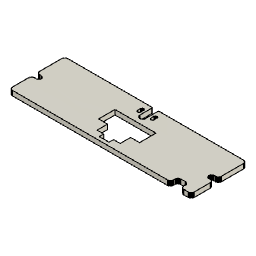
Frame Cover Plate (Autodesk Fusion 360 design; units mm, degrees)
Autodesk Fusion 360 part; units mm, degrees
note: some values were not read from the file. Set by a fixed rule: which sketch regions a step uses.
(part 1 of 3)
sketch "Sketch1" plane through (0, 0, 0) normal (0, 0, 1) x (1, 0, 0) in component "Cover"
  line L0 (69.0119, 5.3264) -> (64.5119, 5.3264)
  line L1 (47.5119, 23.3264) -> (47.5119, 12.3264)
  line L2 (69.0119, 12.3264) -> (69.0119, 5.3264)
  line L3 (75.0119, 12.3264) -> (69.0119, 12.3264)
  line L4 (64.5119, 5.3264) -> (64.5119, 2.3264)
  line L5 (53.5119, 12.3264) -> (53.5119, 5.3264)
  line L6 (64.5119, 2.3264) -> (58.0119, 2.3264)
  line L7 (47.5119, 23.3264) -> (75.0119, 23.3264)
  line L8 (47.5119, 12.3264) -> (53.5119, 12.3264)
  line L9 (58.0119, 2.3264) -> (58.0119, 5.3264)
  line L10 (75.0119, 23.3264) -> (75.0119, 12.3264)
  line L11 (53.5119, 5.3264) -> (58.0119, 5.3264)
  arc A0 (3.7523, 14.957) -> (3.7573, 14.957) centre (3.7548, 14.957) ccw
  arc A1 (3.0339, 14.805) -> (3.0389, 14.805) centre (3.0364, 14.805) ccw
  line L12 (0.8037, 14.387) -> (1.0239, 14.534)
  arc A2 (1.0214, 14.534) -> (1.0264, 14.534) centre (1.0239, 14.534) ccw
  arc A3 (1.0264, 14.534) -> (1.0214, 14.534) centre (1.0239, 14.534) ccw
  line L13 (0.6045, 14.212) -> (0.8037, 14.387)
  arc A4 (1.264, 14.651) -> (1.259, 14.651) centre (1.2615, 14.651) ccw
  arc A5 (0.602, 14.212) -> (0.607, 14.212) centre (0.6045, 14.212) ccw
  line L14 (2.0364, 14.805) -> (3.0364, 14.805)
  arc A6 (1.264, 14.651) -> (1.259, 14.651) centre (1.2615, 14.651) ccw
  arc A7 (0.607, 14.212) -> (0.602, 14.212) centre (0.6045, 14.212) ccw
  arc A8 (2.0339, 14.805) -> (2.0389, 14.805) centre (2.0364, 14.805) ccw
  arc A9 (0.8012, 14.387) -> (0.8062, 14.387) centre (0.8037, 14.387) ccw
  arc A10 (3.043, 14.801) -> (3.048, 14.801) centre (3.0455, 14.801) ccw
  arc A11 (1.5098, 14.736) -> (1.5148, 14.736) centre (1.5123, 14.736) ccw
  line L15 (0.4299, 14.013) -> (0.6045, 14.212)
  arc A12 (0.8012, 14.387) -> (0.8062, 14.387) centre (0.8037, 14.387) ccw
  arc A13 (3.285, 14.818) -> (3.28, 14.818) centre (3.2825, 14.818) ccw
  arc A14 (0.4324, 14.013) -> (0.4274, 14.013) centre (0.4299, 14.013) ccw
  arc A15 (0.8062, 14.387) -> (0.8012, 14.387) centre (0.8037, 14.387) ccw
  arc A16 (0.4274, 14.013) -> (0.4324, 14.013) centre (0.4299, 14.013) ccw
  line L16 (3.5236, 14.871) -> (3.7548, 14.957)
  arc A17 (3.048, 14.801) -> (3.043, 14.801) centre (3.0455, 14.801) ccw
  arc A18 (3.043, 14.801) -> (3.048, 14.801) centre (3.0455, 14.801) ccw
  arc A19 (0.168, 13.555) -> (0.163, 13.555) centre (0.1655, 13.555) ccw
  arc A20 (0.607, 0.598) -> (0.602, 0.598) centre (0.6045, 0.598) ccw
  arc A21 (0.2852, 1.018) -> (0.2802, 1.018) centre (0.2827, 1.018) ccw
  arc A22 (1.7696, 14.788) -> (1.7746, 14.788) centre (1.7721, 14.788) ccw
  arc A23 (3.048, 14.801) -> (3.043, 14.801) centre (3.0455, 14.801) ccw
  arc A24 (0.0089, 12.78) -> (0.0139, 12.78) centre (0.0114, 12.78) ccw
  line L17 (3.7548, 14.957) -> (3.9714, 15.075)
  line L18 (3.2825, 14.818) -> (3.5236, 14.871)
  line L19 (1.0239, 14.534) -> (1.2615, 14.651)
  arc A25 (1.0264, 14.534) -> (1.0214, 14.534) centre (1.0239, 14.534) ccw
  line L20 (3.0455, 14.801) -> (3.2825, 14.818)
  arc A26 (3.0389, 14.805) -> (3.0339, 14.805) centre (3.0364, 14.805) ccw
  arc A27 (3.7573, 14.957) -> (3.7523, 14.957) centre (3.7548, 14.957) ccw
  arc A28 (3.5261, 14.871) -> (3.5211, 14.871) centre (3.5236, 14.871) ccw
  arc A29 (0.4274, 0.797) -> (0.4324, 0.797) centre (0.4299, 0.797) ccw
  arc A30 (4.1714, 15.223) -> (4.1664, 15.223) centre (4.1689, 15.223) ccw
  arc A31 (3.285, 14.818) -> (3.28, 14.818) centre (3.2825, 14.818) ccw
  arc A32 (1.0214, 14.534) -> (1.0264, 14.534) centre (1.0239, 14.534) ccw
  arc A33 (1.7746, 14.788) -> (1.7696, 14.788) centre (1.7721, 14.788) ccw
  arc A34 (0.602, 14.212) -> (0.607, 14.212) centre (0.6045, 14.212) ccw
  arc A35 (0.0262, 13.044) -> (0.0312, 13.044) centre (0.0287, 13.044) ccw
  line L21 (3.0364, 14.805) -> (3.0455, 14.801)
  arc A36 (0.2852, 13.793) -> (0.2802, 13.793) centre (0.2827, 13.793) ccw
  arc A37 (0.163, 13.555) -> (0.168, 13.555) centre (0.1655, 13.555) ccw
  arc A38 (0.4324, 0.797) -> (0.4274, 0.797) centre (0.4299, 0.797) ccw
  arc A39 (3.0339, 14.805) -> (3.0389, 14.805) centre (3.0364, 14.805) ccw
  arc A40 (0.4324, 0.797) -> (0.4274, 0.797) centre (0.4299, 0.797) ccw
  line L22 (0.0114, 2.03) -> (0.0114, 12.78)
  line L23 (0.6045, 0.598) -> (0.8037, 0.423)
  arc A41 (3.9739, 15.075) -> (3.9689, 15.075) centre (3.9714, 15.075) ccw
  arc A42 (3.0389, 14.805) -> (3.0339, 14.805) centre (3.0364, 14.805) ccw
  arc A43 (3.9689, 15.075) -> (3.9739, 15.075) centre (3.9714, 15.075) ccw
  arc A44 (2.0339, 14.805) -> (2.0389, 14.805) centre (2.0364, 14.805) ccw
  arc A45 (3.28, 14.818) -> (3.285, 14.818) centre (3.2825, 14.818) ccw
  line L24 (1.5123, 14.736) -> (1.7721, 14.788)
  arc A46 (2.0389, 14.805) -> (2.0339, 14.805) centre (2.0364, 14.805) ccw
  arc A47 (3.28, 14.818) -> (3.285, 14.818) centre (3.2825, 14.818) ccw
  line L25 (1.7721, 14.788) -> (2.0364, 14.805)
  arc A48 (0.602, 0.598) -> (0.607, 0.598) centre (0.6045, 0.598) ccw
  arc A49 (0.0312, 13.044) -> (0.0262, 13.044) centre (0.0287, 13.044) ccw
  line L26 (0.4299, 0.797) -> (0.6045, 0.598)
  arc A50 (0.168, 1.255) -> (0.163, 1.255) centre (0.1655, 1.255) ccw
  arc A51 (0.607, 14.212) -> (0.602, 14.212) centre (0.6045, 14.212) ccw
  arc A52 (0.0139, 12.78) -> (0.0089, 12.78) centre (0.0114, 12.78) ccw
  arc A53 (0.0779, 1.506) -> (0.0829, 1.506) centre (0.0804, 1.506) ccw
  arc A54 (0.602, 0.598) -> (0.607, 0.598) centre (0.6045, 0.598) ccw
  line L27 (0.1655, 1.255) -> (0.2827, 1.018)
  arc A55 (1.7696, 14.788) -> (1.7746, 14.788) centre (1.7721, 14.788) ccw
  arc A56 (3.5211, 14.871) -> (3.5261, 14.871) centre (3.5236, 14.871) ccw
  arc A57 (1.5148, 14.736) -> (1.5098, 14.736) centre (1.5123, 14.736) ccw
  arc A58 (0.0089, 12.78) -> (0.0139, 12.78) centre (0.0114, 12.78) ccw
  arc A59 (0.4324, 14.013) -> (0.4274, 14.013) centre (0.4299, 14.013) ccw
  line L28 (0.2827, 13.793) -> (0.4299, 14.013)
  arc A60 (3.7523, 14.957) -> (3.7573, 14.957) centre (3.7548, 14.957) ccw
  arc A61 (0.4274, 0.797) -> (0.4324, 0.797) centre (0.4299, 0.797) ccw
  arc A62 (3.5211, 14.871) -> (3.5261, 14.871) centre (3.5236, 14.871) ccw
  arc A63 (3.5261, 14.871) -> (3.5211, 14.871) centre (3.5236, 14.871) ccw
  arc A64 (0.2802, 1.018) -> (0.2852, 1.018) centre (0.2827, 1.018) ccw
  line L29 (1.0239, 0.276) -> (1.2615, 0.159)
  arc A65 (0.0262, 1.766) -> (0.0312, 1.766) centre (0.0287, 1.766) ccw
  line L30 (0.0804, 1.506) -> (0.1655, 1.255)
  arc A66 (106.8089, 0.159) -> (106.8139, 0.159) centre (106.8114, 0.159) ccw
  line L31 (106.8114, 0.159) -> (107.0484, 0.276)
  line L32 (1.7721, 0.022) -> (2.0364, 0.005)
  arc A67 (107.6459, 0.797) -> (107.6409, 0.797) centre (107.6434, 0.797) ccw
  arc A68 (106.8139, 0.159) -> (106.8089, 0.159) centre (106.8114, 0.159) ccw
  arc A69 (1.0214, 0.276) -> (1.0264, 0.276) centre (1.0239, 0.276) ccw
  arc A70 (0.168, 13.555) -> (0.163, 13.555) centre (0.1655, 13.555) ccw
  line L33 (0.0287, 1.766) -> (0.0804, 1.506)
  arc A71 (0.163, 1.255) -> (0.168, 1.255) centre (0.1655, 1.255) ccw
  arc A72 (0.0139, 2.03) -> (0.0089, 2.03) centre (0.0114, 2.03) ccw
  arc A73 (0.168, 1.255) -> (0.163, 1.255) centre (0.1655, 1.255) ccw
  arc A74 (0.0829, 13.304) -> (0.0779, 13.304) centre (0.0804, 13.304) ccw
  arc A75 (0.2802, 13.793) -> (0.2852, 13.793) centre (0.2827, 13.793) ccw
  arc A76 (0.0779, 1.506) -> (0.0829, 1.506) centre (0.0804, 1.506) ccw
  line L34 (0.0114, 12.78) -> (0.0287, 13.044)
  arc A77 (0.163, 1.255) -> (0.168, 1.255) centre (0.1655, 1.255) ccw
  line L35 (0.0287, 13.044) -> (0.0804, 13.304)
  line L36 (0.1655, 13.555) -> (0.2827, 13.793)
  arc A78 (0.0139, 2.03) -> (0.0089, 2.03) centre (0.0114, 2.03) ccw
  arc A79 (0.0312, 13.044) -> (0.0262, 13.044) centre (0.0287, 13.044) ccw
  arc A80 (0.0779, 13.304) -> (0.0829, 13.304) centre (0.0804, 13.304) ccw
  arc A81 (0.0312, 1.766) -> (0.0262, 1.766) centre (0.0287, 1.766) ccw
  arc A82 (0.0312, 1.766) -> (0.0262, 1.766) centre (0.0287, 1.766) ccw
  line L37 (0.2827, 1.018) -> (0.4299, 0.797)
  arc A83 (0.0089, 2.03) -> (0.0139, 2.03) centre (0.0114, 2.03) ccw
  arc A84 (0.2802, 13.793) -> (0.2852, 13.793) centre (0.2827, 13.793) ccw
  arc A85 (107.4709, 0.598) -> (107.4659, 0.598) centre (107.4684, 0.598) ccw
  arc A86 (1.0264, 0.276) -> (1.0214, 0.276) centre (1.0239, 0.276) ccw
  arc A87 (2.0389, 0.005) -> (2.0339, 0.005) centre (2.0364, 0.005) ccw
  arc A88 (0.2852, 1.018) -> (0.2802, 1.018) centre (0.2827, 1.018) ccw
  arc A89 (0.0829, 1.506) -> (0.0779, 1.506) centre (0.0804, 1.506) ccw
  arc A90 (0.8012, 0.423) -> (0.8062, 0.423) centre (0.8037, 0.423) ccw
  arc A91 (1.7696, 0.022) -> (1.7746, 0.022) centre (1.7721, 0.022) ccw
  arc A92 (0.2852, 13.793) -> (0.2802, 13.793) centre (0.2827, 13.793) ccw
  arc A93 (106.2979, 0.022) -> (106.3029, 0.022) centre (106.3004, 0.022) ccw
  arc A94 (1.264, 0.159) -> (1.259, 0.159) centre (1.2615, 0.159) ccw
  arc A95 (1.5098, 0.074) -> (1.5148, 0.074) centre (1.5123, 0.074) ccw
  line L38 (107.6434, 0.797) -> (107.7904, 1.018)
  arc A96 (1.7746, 0.022) -> (1.7696, 0.022) centre (1.7721, 0.022) ccw
  arc A97 (0.0262, 13.044) -> (0.0312, 13.044) centre (0.0287, 13.044) ccw
  arc A98 (0.0139, 12.78) -> (0.0089, 12.78) centre (0.0114, 12.78) ccw
  line L39 (0.0114, 2.03) -> (0.0287, 1.766)
  arc A99 (0.0829, 13.304) -> (0.0779, 13.304) centre (0.0804, 13.304) ccw
  arc A100 (0.0089, 2.03) -> (0.0139, 2.03) centre (0.0114, 2.03) ccw
  line L40 (1.5123, 0.074) -> (1.7721, 0.022)
  arc A101 (0.163, 13.555) -> (0.168, 13.555) centre (0.1655, 13.555) ccw
  arc A102 (0.4274, 14.013) -> (0.4324, 14.013) centre (0.4299, 14.013) ccw
  arc A103 (106.3029, 0.022) -> (106.2979, 0.022) centre (106.3004, 0.022) ccw
  arc A104 (106.5579, 0.074) -> (106.5629, 0.074) centre (106.5604, 0.074) ccw
  arc A105 (0.0779, 13.304) -> (0.0829, 13.304) centre (0.0804, 13.304) ccw
  arc A106 (1.259, 0.159) -> (1.264, 0.159) centre (1.2615, 0.159) ccw
  arc A107 (1.0264, 0.276) -> (1.0214, 0.276) centre (1.0239, 0.276) ccw
  arc A108 (1.5148, 0.074) -> (1.5098, 0.074) centre (1.5123, 0.074) ccw
  arc A109 (106.8089, 0.159) -> (106.8139, 0.159) centre (106.8114, 0.159) ccw
  arc A110 (0.2802, 1.018) -> (0.2852, 1.018) centre (0.2827, 1.018) ccw
  line L41 (0.0804, 13.304) -> (0.1655, 13.555)
  arc A111 (0.0829, 1.506) -> (0.0779, 1.506) centre (0.0804, 1.506) ccw
  arc A112 (0.0262, 1.766) -> (0.0312, 1.766) centre (0.0287, 1.766) ccw
  arc A113 (106.0389, 0.005) -> (106.0339, 0.005) centre (106.0364, 0.005) ccw
  arc A114 (1.7746, 0.022) -> (1.7696, 0.022) centre (1.7721, 0.022) ccw
  line L42 (2.0364, 0.005) -> (106.0364, 0.005)
  line L43 (108.0444, 1.766) -> (108.0614, 2.03)
  line L44 (108.0574, 3.039) -> (108.0744, 3.288)
  arc A115 (108.2049, 3.787) -> (108.2099, 3.787) centre (108.2074, 3.787) ccw
  arc A116 (0.8012, 0.423) -> (0.8062, 0.423) centre (0.8037, 0.423) ccw
  arc A117 (107.6459, 0.797) -> (107.6409, 0.797) centre (107.6434, 0.797) ccw
  line L45 (106.0364, 0.005) -> (106.3004, 0.022)
  line L46 (107.2694, 0.423) -> (107.4684, 0.598)
  arc A118 (2.0389, 0.005) -> (2.0339, 0.005) centre (2.0364, 0.005) ccw
  arc A119 (106.8139, 0.159) -> (106.8089, 0.159) centre (106.8114, 0.159) ccw
  arc A120 (107.0459, 0.276) -> (107.0509, 0.276) centre (107.0484, 0.276) ccw
  line L47 (106.5604, 0.074) -> (106.8114, 0.159)
  arc A121 (107.4709, 0.598) -> (107.4659, 0.598) centre (107.4684, 0.598) ccw
  arc A122 (107.2719, 0.423) -> (107.2669, 0.423) centre (107.2694, 0.423) ccw
  arc A123 (106.0389, 0.005) -> (106.0339, 0.005) centre (106.0364, 0.005) ccw
  arc A124 (1.5148, 0.074) -> (1.5098, 0.074) centre (1.5123, 0.074) ccw
  line L48 (106.3004, 0.022) -> (106.5604, 0.074)
  arc A125 (107.2669, 0.423) -> (107.2719, 0.423) centre (107.2694, 0.423) ccw
  line L49 (0.8037, 0.423) -> (1.0239, 0.276)
  arc A126 (107.9949, 1.506) -> (107.9899, 1.506) centre (107.9924, 1.506) ccw
  arc A127 (108.1269, 3.542) -> (108.1219, 3.542) centre (108.1244, 3.542) ccw
  arc A128 (1.5098, 0.074) -> (1.5148, 0.074) centre (1.5123, 0.074) ccw
  arc A129 (0.607, 0.598) -> (0.602, 0.598) centre (0.6045, 0.598) ccw
  arc A130 (107.4659, 0.598) -> (107.4709, 0.598) centre (107.4684, 0.598) ccw
  arc A131 (106.2979, 0.022) -> (106.3029, 0.022) centre (106.3004, 0.022) ccw
  arc A132 (106.5629, 0.074) -> (106.5579, 0.074) centre (106.5604, 0.074) ccw
  arc A133 (107.6409, 0.797) -> (107.6459, 0.797) centre (107.6434, 0.797) ccw
  line L50 (1.2615, 0.159) -> (1.5123, 0.074)
  arc A134 (1.259, 0.159) -> (1.264, 0.159) centre (1.2615, 0.159) ccw
  arc A135 (0.8062, 0.423) -> (0.8012, 0.423) centre (0.8037, 0.423) ccw
  arc A136 (0.8062, 0.423) -> (0.8012, 0.423) centre (0.8037, 0.423) ccw
  arc A137 (108.0599, 3.039) -> (108.0549, 3.039) centre (108.0574, 3.039) ccw
  arc A138 (1.7696, 0.022) -> (1.7746, 0.022) centre (1.7721, 0.022) ccw
  arc A139 (2.0339, 0.005) -> (2.0389, 0.005) centre (2.0364, 0.005) ccw
  line L51 (107.4684, 0.598) -> (107.6434, 0.797)
  arc A140 (106.3029, 0.022) -> (106.2979, 0.022) centre (106.3004, 0.022) ccw
  arc A141 (106.5629, 0.074) -> (106.5579, 0.074) centre (106.5604, 0.074) ccw
  arc A142 (107.6409, 0.797) -> (107.6459, 0.797) centre (107.6434, 0.797) ccw
  arc A143 (1.0214, 0.276) -> (1.0264, 0.276) centre (1.0239, 0.276) ccw
  arc A144 (108.0469, 1.766) -> (108.0419, 1.766) centre (108.0444, 1.766) ccw
  line L52 (108.0574, 3.039) -> (108.0614, 3.03)
  arc A145 (106.0339, 0.005) -> (106.0389, 0.005) centre (106.0364, 0.005) ccw
  arc A146 (106.5579, 0.074) -> (106.5629, 0.074) centre (106.5604, 0.074) ccw
  arc A147 (108.0719, 3.288) -> (108.0769, 3.288) centre (108.0744, 3.288) ccw
  arc A148 (108.2099, 3.787) -> (108.2049, 3.787) centre (108.2074, 3.787) ccw
  arc A149 (107.4659, 0.598) -> (107.4709, 0.598) centre (107.4684, 0.598) ccw
  arc A150 (107.7879, 1.018) -> (107.7929, 1.018) centre (107.7904, 1.018) ccw
  arc A151 (108.0469, 1.766) -> (108.0419, 1.766) centre (108.0444, 1.766) ccw
  arc A152 (108.0719, 3.288) -> (108.0769, 3.288) centre (108.0744, 3.288) ccw
  arc A153 (106.0339, 0.005) -> (106.0389, 0.005) centre (106.0364, 0.005) ccw
  arc A154 (107.0509, 0.276) -> (107.0459, 0.276) centre (107.0484, 0.276) ccw
  arc A155 (1.264, 0.159) -> (1.259, 0.159) centre (1.2615, 0.159) ccw
  arc A156 (2.0339, 0.005) -> (2.0389, 0.005) centre (2.0364, 0.005) ccw
  arc A157 (65.9959, 29.6125) -> (65.9909, 29.6125) centre (65.9934, 29.6125) ccw
  arc A158 (64.5779, 30.1597) -> (64.5829, 30.1597) centre (64.5804, 30.1597) ccw
  line L53 (65.6314, 29.5094) -> (65.8174, 29.5441)
  arc A159 (65.9909, 29.6125) -> (65.9959, 29.6125) centre (65.9934, 29.6125) ccw
  arc A160 (64.5829, 30.1597) -> (64.5779, 30.1597) centre (64.5804, 30.1597) ccw
  arc A161 (64.7819, 29.8395) -> (64.7769, 29.8395) centre (64.7794, 29.8395) ccw
  line L54 (64.5114, 32.53) -> (64.5284, 32.7183)
  arc A162 (64.5089, 32.53) -> (64.5139, 32.53) centre (64.5114, 32.53) ccw
  arc A163 (64.5139, 32.53) -> (64.5089, 32.53) centre (64.5114, 32.53) ccw
  arc A164 (64.5259, 32.7183) -> (64.5309, 32.7183) centre (64.5284, 32.7183) ccw
  arc A165 (64.5829, 32.9003) -> (64.5779, 32.9003) centre (64.5804, 32.9003) ccw
  arc A166 (64.5259, 30.3417) -> (64.5309, 30.3417) centre (64.5284, 30.3417) ccw
  line L55 (64.7794, 29.8395) -> (64.9184, 29.712)
  arc A167 (64.5089, 30.53) -> (64.5139, 30.53) centre (64.5114, 30.53) ccw
  line L56 (65.0794, 29.6125) -> (65.2554, 29.5441)
  line L57 (65.8174, 29.5441) -> (65.9934, 29.6125)
  line L58 (64.5114, 30.53) -> (64.5284, 30.3417)
  arc A168 (65.9909, 29.6125) -> (65.9959, 29.6125) centre (65.9934, 29.6125) ccw
  arc A169 (64.5259, 30.3417) -> (64.5309, 30.3417) centre (64.5284, 30.3417) ccw
  arc A170 (66.5419, 32.7183) -> (66.5469, 32.7183) centre (66.5444, 32.7183) ccw
  arc A171 (65.8199, 29.5441) -> (65.8149, 29.5441) centre (65.8174, 29.5441) ccw
  arc A172 (66.1519, 29.712) -> (66.1569, 29.712) centre (66.1544, 29.712) ccw
  arc A173 (65.6339, 29.5094) -> (65.6289, 29.5094) centre (65.6314, 29.5094) ccw
  line L59 (64.9184, 29.712) -> (65.0794, 29.6125)
  arc A174 (65.6339, 29.5094) -> (65.6289, 29.5094) centre (65.6314, 29.5094) ccw
  arc A175 (65.4389, 29.5094) -> (65.4439, 29.5094) centre (65.4414, 29.5094) ccw
  arc A176 (65.0819, 29.6125) -> (65.0769, 29.6125) centre (65.0794, 29.6125) ccw
  arc A177 (64.5089, 32.53) -> (64.5139, 32.53) centre (64.5114, 32.53) ccw
  line L60 (65.9934, 29.6125) -> (66.1544, 29.712)
  arc A178 (65.9959, 29.6125) -> (65.9909, 29.6125) centre (65.9934, 29.6125) ccw
  arc A179 (65.0769, 29.6125) -> (65.0819, 29.6125) centre (65.0794, 29.6125) ccw
  arc A180 (64.9159, 29.712) -> (64.9209, 29.712) centre (64.9184, 29.712) ccw
  arc A181 (64.6679, 29.9904) -> (64.6629, 29.9904) centre (64.6654, 29.9904) ccw
  arc A182 (65.8149, 29.5441) -> (65.8199, 29.5441) centre (65.8174, 29.5441) ccw
  arc A183 (64.5139, 30.53) -> (64.5089, 30.53) centre (64.5114, 30.53) ccw
  arc A184 (64.6629, 29.9904) -> (64.6679, 29.9904) centre (64.6654, 29.9904) ccw
  arc A185 (65.4439, 29.5094) -> (65.4389, 29.5094) centre (65.4414, 29.5094) ccw
  arc A186 (65.8149, 29.5441) -> (65.8199, 29.5441) centre (65.8174, 29.5441) ccw
  arc A187 (64.9209, 29.712) -> (64.9159, 29.712) centre (64.9184, 29.712) ccw
  arc A188 (66.1519, 33.348) -> (66.1569, 33.348) centre (66.1544, 33.348) ccw
  arc A189 (66.5589, 30.53) -> (66.5639, 30.53) centre (66.5614, 30.53) ccw
  arc A190 (66.4949, 32.9003) -> (66.4899, 32.9003) centre (66.4924, 32.9003) ccw
  arc A191 (66.2959, 29.8395) -> (66.2909, 29.8395) centre (66.2934, 29.8395) ccw
  line L61 (66.4924, 30.1597) -> (66.5444, 30.3417)
  line L62 (65.2554, 29.5441) -> (65.4414, 29.5094)
  arc A192 (64.5309, 30.3417) -> (64.5259, 30.3417) centre (64.5284, 30.3417) ccw
  arc A193 (66.1569, 29.712) -> (66.1519, 29.712) centre (66.1544, 29.712) ccw
  arc A194 (65.0819, 29.6125) -> (65.0769, 29.6125) centre (65.0794, 29.6125) ccw
  arc A195 (64.7769, 29.8395) -> (64.7819, 29.8395) centre (64.7794, 29.8395) ccw
  arc A196 (65.4439, 29.5094) -> (65.4389, 29.5094) centre (65.4414, 29.5094) ccw
  arc A197 (65.2579, 29.5441) -> (65.2529, 29.5441) centre (65.2554, 29.5441) ccw
  arc A198 (65.0769, 29.6125) -> (65.0819, 29.6125) centre (65.0794, 29.6125) ccw
  arc A199 (64.6629, 29.9904) -> (64.6679, 29.9904) centre (64.6654, 29.9904) ccw
  arc A200 (65.6289, 29.5094) -> (65.6339, 29.5094) centre (65.6314, 29.5094) ccw
  line L63 (64.5804, 30.1597) -> (64.6654, 29.9904)
  line L64 (66.1544, 29.712) -> (66.2934, 29.8395)
  arc A201 (64.5139, 32.53) -> (64.5089, 32.53) centre (64.5114, 32.53) ccw
  line L65 (65.4414, 29.5094) -> (65.6314, 29.5094)
  arc A202 (65.4389, 29.5094) -> (65.4439, 29.5094) centre (65.4414, 29.5094) ccw
  line L66 (64.6654, 29.9904) -> (64.7794, 29.8395)
  arc A203 (64.7819, 29.8395) -> (64.7769, 29.8395) centre (64.7794, 29.8395) ccw
  arc A204 (66.1519, 29.712) -> (66.1569, 29.712) centre (66.1544, 29.712) ccw
  arc A205 (64.5309, 30.3417) -> (64.5259, 30.3417) centre (64.5284, 30.3417) ccw
  arc A206 (65.6289, 29.5094) -> (65.6339, 29.5094) centre (65.6314, 29.5094) ccw
  arc A207 (64.7769, 29.8395) -> (64.7819, 29.8395) centre (64.7794, 29.8395) ccw
  arc A208 (64.5829, 30.1597) -> (64.5779, 30.1597) centre (64.5804, 30.1597) ccw
  arc A209 (65.2529, 29.5441) -> (65.2579, 29.5441) centre (65.2554, 29.5441) ccw
  arc A210 (64.5779, 30.1597) -> (64.5829, 30.1597) centre (64.5804, 30.1597) ccw
  arc A211 (65.8199, 29.5441) -> (65.8149, 29.5441) centre (65.8174, 29.5441) ccw
  arc A212 (64.6679, 29.9904) -> (64.6629, 29.9904) centre (64.6654, 29.9904) ccw
  arc A213 (65.2529, 29.5441) -> (65.2579, 29.5441) centre (65.2554, 29.5441) ccw
  arc A214 (65.2579, 29.5441) -> (65.2529, 29.5441) centre (65.2554, 29.5441) ccw
  arc A215 (64.9209, 29.712) -> (64.9159, 29.712) centre (64.9184, 29.712) ccw
  line L67 (64.5284, 30.3417) -> (64.5804, 30.1597)
  arc A216 (64.9159, 29.712) -> (64.9209, 29.712) centre (64.9184, 29.712) ccw
  arc A217 (65.9959, 33.4475) -> (65.9909, 33.4475) centre (65.9934, 33.4475) ccw
  arc A218 (66.5639, 30.53) -> (66.5589, 30.53) centre (66.5614, 30.53) ccw
  arc A219 (66.1569, 33.348) -> (66.1519, 33.348) centre (66.1544, 33.348) ccw
  arc A220 (66.2959, 33.2205) -> (66.2909, 33.2205) centre (66.2934, 33.2205) ccw
  arc A221 (65.8199, 33.5159) -> (65.8149, 33.5159) centre (65.8174, 33.5159) ccw
  arc A222 (66.4049, 33.0696) -> (66.4099, 33.0696) centre (66.4074, 33.0696) ccw
  arc A223 (66.2959, 29.8395) -> (66.2909, 29.8395) centre (66.2934, 29.8395) ccw
  arc A224 (66.5589, 30.53) -> (66.5639, 30.53) centre (66.5614, 30.53) ccw
  arc A225 (66.5469, 32.7183) -> (66.5419, 32.7183) centre (66.5444, 32.7183) ccw
  line L68 (65.8174, 33.5159) -> (65.9934, 33.4475)
  arc A226 (66.5589, 32.53) -> (66.5639, 32.53) centre (66.5614, 32.53) ccw
  arc A227 (66.2909, 29.8395) -> (66.2959, 29.8395) centre (66.2934, 29.8395) ccw
  arc A228 (66.4949, 30.1597) -> (66.4899, 30.1597) centre (66.4924, 30.1597) ccw
  arc A229 (66.4949, 30.1597) -> (66.4899, 30.1597) centre (66.4924, 30.1597) ccw
  line L69 (66.5614, 30.53) -> (66.5614, 32.53)
  arc A230 (66.4099, 29.9904) -> (66.4049, 29.9904) centre (66.4074, 29.9904) ccw
  arc A231 (66.2909, 33.2205) -> (66.2959, 33.2205) centre (66.2934, 33.2205) ccw
  line L70 (66.5444, 32.7183) -> (66.5614, 32.53)
  arc A232 (66.5469, 30.3417) -> (66.5419, 30.3417) centre (66.5444, 30.3417) ccw
  arc A233 (66.5419, 30.3417) -> (66.5469, 30.3417) centre (66.5444, 30.3417) ccw
  arc A234 (66.4099, 33.0696) -> (66.4049, 33.0696) centre (66.4074, 33.0696) ccw
  arc A235 (66.5589, 32.53) -> (66.5639, 32.53) centre (66.5614, 32.53) ccw
  arc A236 (66.5469, 32.7183) -> (66.5419, 32.7183) centre (66.5444, 32.7183) ccw
  line L71 (66.1544, 33.348) -> (66.2934, 33.2205)
  arc A237 (120.0389, 37.055) -> (120.0339, 37.055) centre (120.0364, 37.055) ccw
  arc A238 (66.4899, 30.1597) -> (66.4949, 30.1597) centre (66.4924, 30.1597) ccw
  arc A239 (65.8149, 33.5159) -> (65.8199, 33.5159) centre (65.8174, 33.5159) ccw
  arc A240 (66.4049, 29.9904) -> (66.4099, 29.9904) centre (66.4074, 29.9904) ccw
  arc A241 (66.5639, 30.53) -> (66.5589, 30.53) centre (66.5614, 30.53) ccw
  arc A242 (65.9909, 33.4475) -> (65.9959, 33.4475) centre (65.9934, 33.4475) ccw
  line L72 (66.4074, 33.0696) -> (66.4924, 32.9003)
  arc A243 (66.4099, 33.0696) -> (66.4049, 33.0696) centre (66.4074, 33.0696) ccw
  arc A244 (66.5639, 32.53) -> (66.5589, 32.53) centre (66.5614, 32.53) ccw
  arc A245 (66.4899, 32.9003) -> (66.4949, 32.9003) centre (66.4924, 32.9003) ccw
  line L73 (66.5444, 30.3417) -> (66.5614, 30.53)
  arc A246 (66.5419, 32.7183) -> (66.5469, 32.7183) centre (66.5444, 32.7183) ccw
  arc A247 (65.9909, 33.4475) -> (65.9959, 33.4475) centre (65.9934, 33.4475) ccw
  arc A248 (66.5469, 30.3417) -> (66.5419, 30.3417) centre (66.5444, 30.3417) ccw
  arc A249 (66.1519, 33.348) -> (66.1569, 33.348) centre (66.1544, 33.348) ccw
  line L74 (65.9934, 33.4475) -> (66.1544, 33.348)
  arc A250 (66.5639, 32.53) -> (66.5589, 32.53) centre (66.5614, 32.53) ccw
  line L75 (66.4924, 32.9003) -> (66.5444, 32.7183)
  line L76 (66.2934, 33.2205) -> (66.4074, 33.0696)
  arc A251 (66.4949, 32.9003) -> (66.4899, 32.9003) centre (66.4924, 32.9003) ccw
  arc A252 (66.4899, 32.9003) -> (66.4949, 32.9003) centre (66.4924, 32.9003) ccw
  arc A253 (66.4899, 30.1597) -> (66.4949, 30.1597) centre (66.4924, 30.1597) ccw
  arc A254 (66.1569, 29.712) -> (66.1519, 29.712) centre (66.1544, 29.712) ccw
  arc A255 (66.2909, 29.8395) -> (66.2959, 29.8395) centre (66.2934, 29.8395) ccw
  line L77 (66.4074, 29.9904) -> (66.4924, 30.1597)
  arc A256 (66.4099, 29.9904) -> (66.4049, 29.9904) centre (66.4074, 29.9904) ccw
  arc A257 (66.4049, 29.9904) -> (66.4099, 29.9904) centre (66.4074, 29.9904) ccw
  arc A258 (66.1569, 33.348) -> (66.1519, 33.348) centre (66.1544, 33.348) ccw
  arc A259 (66.2959, 33.2205) -> (66.2909, 33.2205) centre (66.2934, 33.2205) ccw
  arc A260 (66.5419, 30.3417) -> (66.5469, 30.3417) centre (66.5444, 30.3417) ccw
  line L78 (66.2934, 29.8395) -> (66.4074, 29.9904)
  arc A261 (65.9959, 33.4475) -> (65.9909, 33.4475) centre (65.9934, 33.4475) ccw
  arc A262 (66.4049, 33.0696) -> (66.4099, 33.0696) centre (66.4074, 33.0696) ccw
  arc A263 (66.2909, 33.2205) -> (66.2959, 33.2205) centre (66.2934, 33.2205) ccw
  line L79 (120.3004, 37.0377) -> (120.5604, 36.986)
  arc A264 (120.2979, 37.0377) -> (120.3029, 37.0377) centre (120.3004, 37.0377) ccw
  arc A265 (63.2069, 36.9405) -> (63.2119, 36.9405) centre (63.2094, 36.9405) ccw
  arc A266 (120.5629, 36.986) -> (120.5579, 36.986) centre (120.5604, 36.986) ccw
  line L80 (120.0364, 37.055) -> (120.3004, 37.0377)
  line L81 (63.3084, 37.003) -> (63.4194, 37.0418)
  arc A267 (62.9999, 28.2604) -> (62.9949, 28.2604) centre (62.9974, 28.2604) ccw
  arc A268 (63.0089, 36.53) -> (63.0139, 36.53) centre (63.0114, 36.53) ccw
  arc A269 (62.9949, 28.2604) -> (62.9999, 28.2604) centre (62.9974, 28.2604) ccw
  line L82 (62.9974, 28.2604) -> (63.0154, 28.5204)
  arc A270 (120.0339, 37.055) -> (120.0389, 37.055) centre (120.0364, 37.055) ccw
  arc A271 (63.1239, 36.8573) -> (63.1289, 36.8573) centre (63.1264, 36.8573) ccw
  arc A272 (63.0129, 28.5204) -> (63.0179, 28.5204) centre (63.0154, 28.5204) ccw
  arc A273 (63.0269, 36.6468) -> (63.0219, 36.6468) centre (63.0244, 36.6468) ccw
  arc A274 (63.0129, 28.5204) -> (63.0179, 28.5204) centre (63.0154, 28.5204) ccw
  arc A275 (63.3059, 37.003) -> (63.3109, 37.003) centre (63.3084, 37.003) ccw
  arc A276 (63.0179, 28.5204) -> (63.0129, 28.5204) centre (63.0154, 28.5204) ccw
  arc A277 (63.4169, 37.0418) -> (63.4219, 37.0418) centre (63.4194, 37.0418) ccw
  arc A278 (63.0089, 36.53) -> (63.0139, 36.53) centre (63.0114, 36.53) ccw
  arc A279 (63.2119, 36.9405) -> (63.2069, 36.9405) centre (63.2094, 36.9405) ccw
  arc A280 (120.3029, 37.0377) -> (120.2979, 37.0377) centre (120.3004, 37.0377) ccw
  line L83 (63.0114, 28.53) -> (63.0114, 36.53)
  arc A281 (63.2119, 36.9405) -> (63.2069, 36.9405) centre (63.2094, 36.9405) ccw
  arc A282 (120.3029, 37.0377) -> (120.2979, 37.0377) centre (120.3004, 37.0377) ccw
  arc A283 (63.1289, 36.8573) -> (63.1239, 36.8573) centre (63.1264, 36.8573) ccw
  arc A284 (63.0659, 36.7578) -> (63.0609, 36.7578) centre (63.0634, 36.7578) ccw
  arc A285 (63.0269, 36.6468) -> (63.0219, 36.6468) centre (63.0244, 36.6468) ccw
  arc A286 (63.0089, 28.53) -> (63.0139, 28.53) centre (63.0114, 28.53) ccw
  arc A287 (120.0389, 37.055) -> (120.0339, 37.055) centre (120.0364, 37.055) ccw
  line L84 (63.0114, 28.53) -> (63.0154, 28.5204)
  arc A288 (63.4219, 37.0418) -> (63.4169, 37.0418) centre (63.4194, 37.0418) ccw
  arc A289 (63.5389, 37.055) -> (63.5339, 37.055) centre (63.5364, 37.055) ccw
  arc A290 (63.2069, 36.9405) -> (63.2119, 36.9405) centre (63.2094, 36.9405) ccw
  arc A291 (63.0609, 36.7578) -> (63.0659, 36.7578) centre (63.0634, 36.7578) ccw
  arc A292 (63.4219, 37.0418) -> (63.4169, 37.0418) centre (63.4194, 37.0418) ccw
  arc A293 (63.0089, 28.53) -> (63.0139, 28.53) centre (63.0114, 28.53) ccw
  line L85 (63.2094, 36.9405) -> (63.3084, 37.003)
  arc A294 (63.5339, 37.055) -> (63.5389, 37.055) centre (63.5364, 37.055) ccw
  arc A295 (63.0219, 36.6468) -> (63.0269, 36.6468) centre (63.0244, 36.6468) ccw
  arc A296 (63.1239, 36.8573) -> (63.1289, 36.8573) centre (63.1264, 36.8573) ccw
  line L86 (63.5364, 37.055) -> (120.0364, 37.055)
  arc A297 (63.4169, 37.0418) -> (63.4219, 37.0418) centre (63.4194, 37.0418) ccw
  arc A298 (63.0179, 28.5204) -> (63.0129, 28.5204) centre (63.0154, 28.5204) ccw
  arc A299 (63.5389, 37.055) -> (63.5339, 37.055) centre (63.5364, 37.055) ccw
  arc A300 (63.3109, 37.003) -> (63.3059, 37.003) centre (63.3084, 37.003) ccw
  arc A301 (63.0609, 36.7578) -> (63.0659, 36.7578) centre (63.0634, 36.7578) ccw
  line L87 (63.4194, 37.0418) -> (63.5364, 37.055)
  arc A302 (63.0139, 36.53) -> (63.0089, 36.53) centre (63.0114, 36.53) ccw
  arc A303 (63.1289, 36.8573) -> (63.1239, 36.8573) centre (63.1264, 36.8573) ccw
  line L88 (63.0634, 36.7578) -> (63.1264, 36.8573)
  arc A304 (63.0219, 36.6468) -> (63.0269, 36.6468) centre (63.0244, 36.6468) ccw
  line L89 (63.0114, 36.53) -> (63.0244, 36.6468)
  line L90 (63.1264, 36.8573) -> (63.2094, 36.9405)
  arc A305 (63.3109, 37.003) -> (63.3059, 37.003) centre (63.3084, 37.003) ccw
  line L91 (63.0244, 36.6468) -> (63.0634, 36.7578)
  arc A306 (63.0139, 28.53) -> (63.0089, 28.53) centre (63.0114, 28.53) ccw
  arc A307 (63.0659, 36.7578) -> (63.0609, 36.7578) centre (63.0634, 36.7578) ccw
  arc A308 (63.0139, 36.53) -> (63.0089, 36.53) centre (63.0114, 36.53) ccw
  arc A309 (63.0139, 28.53) -> (63.0089, 28.53) centre (63.0114, 28.53) ccw
  arc A310 (120.5579, 36.986) -> (120.5629, 36.986) centre (120.5604, 36.986) ccw
  arc A311 (120.2979, 37.0377) -> (120.3029, 37.0377) centre (120.3004, 37.0377) ccw
  arc A312 (63.5339, 37.055) -> (63.5389, 37.055) centre (63.5364, 37.055) ccw
  arc A313 (63.3059, 37.003) -> (63.3109, 37.003) centre (63.3084, 37.003) ccw
  arc A314 (61.9449, 26.7723) -> (61.9499, 26.7723) centre (61.9474, 26.7723) ccw
  line L92 (62.7274, 27.5014) -> (62.8524, 27.7413)
  line L93 (61.4394, 26.5918) -> (61.6994, 26.6647)
  arc A315 (61.4419, 26.5918) -> (61.4369, 26.5918) centre (61.4394, 26.5918) ccw
  line L94 (62.5724, 27.2807) -> (62.7274, 27.5014)
  arc A316 (60.9038, 26.555) -> (60.8988, 26.555) centre (60.9013, 26.555) ccw
  arc A317 (60.376, 26.6647) -> (60.371, 26.6647) centre (60.3735, 26.6647) ccw
  arc A318 (62.1759, 26.9127) -> (62.1809, 26.9127) centre (62.1784, 26.9127) ccw
  arc A319 (61.1689, 26.555) -> (61.1739, 26.555) centre (61.1714, 26.555) ccw
  arc A320 (61.7019, 26.6647) -> (61.6969, 26.6647) centre (61.6994, 26.6647) ccw
  arc A321 (120.0339, 37.055) -> (120.0389, 37.055) centre (120.0364, 37.055) ccw
  arc A322 (62.8499, 27.7413) -> (62.8549, 27.7413) centre (62.8524, 27.7413) ccw
  arc A323 (61.4369, 26.5918) -> (61.4419, 26.5918) centre (61.4394, 26.5918) ccw
  arc A324 (61.1739, 26.555) -> (61.1689, 26.555) centre (61.1714, 26.555) ccw
  arc A325 (61.4419, 26.5918) -> (61.4369, 26.5918) centre (61.4394, 26.5918) ccw
  arc A326 (62.3899, 27.0832) -> (62.3849, 27.0832) centre (62.3874, 27.0832) ccw
  arc A327 (62.9999, 28.2604) -> (62.9949, 28.2604) centre (62.9974, 28.2604) ccw
  arc A328 (62.7299, 27.5014) -> (62.7249, 27.5014) centre (62.7274, 27.5014) ccw
  arc A329 (61.9499, 26.7723) -> (61.9449, 26.7723) centre (61.9474, 26.7723) ccw
  arc A330 (61.1689, 26.555) -> (61.1739, 26.555) centre (61.1714, 26.555) ccw
  arc A331 (62.1809, 26.9127) -> (62.1759, 26.9127) centre (62.1784, 26.9127) ccw
  arc A332 (60.371, 26.6647) -> (60.376, 26.6647) centre (60.3735, 26.6647) ccw
  arc A333 (62.5699, 27.2807) -> (62.5749, 27.2807) centre (62.5724, 27.2807) ccw
  arc A334 (60.8988, 26.555) -> (60.9038, 26.555) centre (60.9013, 26.555) ccw
  arc A335 (60.6311, 26.5918) -> (60.6361, 26.5918) centre (60.6336, 26.5918) ccw
  arc A336 (62.9949, 28.2604) -> (62.9999, 28.2604) centre (62.9974, 28.2604) ccw
  arc A337 (61.1739, 26.555) -> (61.1689, 26.555) centre (61.1714, 26.555) ccw
  line L95 (60.9013, 26.555) -> (61.1714, 26.555)
  arc A338 (62.8499, 27.7413) -> (62.8549, 27.7413) centre (62.8524, 27.7413) ccw
  arc A339 (60.8988, 26.555) -> (60.9038, 26.555) centre (60.9013, 26.555) ccw
  arc A340 (62.1809, 26.9127) -> (62.1759, 26.9127) centre (62.1784, 26.9127) ccw
  arc A341 (62.3849, 27.0832) -> (62.3899, 27.0832) centre (62.3874, 27.0832) ccw
  arc A342 (62.7249, 27.5014) -> (62.7299, 27.5014) centre (62.7274, 27.5014) ccw
  arc A343 (62.3899, 27.0832) -> (62.3849, 27.0832) centre (62.3874, 27.0832) ccw
  arc A344 (62.9399, 27.9959) -> (62.9449, 27.9959) centre (62.9424, 27.9959) ccw
  line L96 (60.3735, 26.6647) -> (60.6336, 26.5918)
  arc A345 (60.6311, 26.5918) -> (60.6361, 26.5918) centre (60.6336, 26.5918) ccw
  line L97 (62.3874, 27.0832) -> (62.5724, 27.2807)
  arc A346 (61.4369, 26.5918) -> (61.4419, 26.5918) centre (61.4394, 26.5918) ccw
  line L98 (62.9424, 27.9959) -> (62.9974, 28.2604)
  line L99 (62.1784, 26.9127) -> (62.3874, 27.0832)
  arc A347 (62.5749, 27.2807) -> (62.5699, 27.2807) centre (62.5724, 27.2807) ccw
  line L100 (61.9474, 26.7723) -> (62.1784, 26.9127)
  arc A348 (62.5699, 27.2807) -> (62.5749, 27.2807) centre (62.5724, 27.2807) ccw
  arc A349 (61.6969, 26.6647) -> (61.7019, 26.6647) centre (61.6994, 26.6647) ccw
  arc A350 (61.7019, 26.6647) -> (61.6969, 26.6647) centre (61.6994, 26.6647) ccw
  line L101 (62.8524, 27.7413) -> (62.9424, 27.9959)
  arc A351 (62.3849, 27.0832) -> (62.3899, 27.0832) centre (62.3874, 27.0832) ccw
  arc A352 (60.6361, 26.5918) -> (60.6311, 26.5918) centre (60.6336, 26.5918) ccw
  arc A353 (61.6969, 26.6647) -> (61.7019, 26.6647) centre (61.6994, 26.6647) ccw
  arc A354 (61.9449, 26.7723) -> (61.9499, 26.7723) centre (61.9474, 26.7723) ccw
  arc A355 (62.5749, 27.2807) -> (62.5699, 27.2807) centre (62.5724, 27.2807) ccw
  arc A356 (62.7299, 27.5014) -> (62.7249, 27.5014) centre (62.7274, 27.5014) ccw
  arc A357 (62.8549, 27.7413) -> (62.8499, 27.7413) centre (62.8524, 27.7413) ccw
  line L102 (60.6336, 26.5918) -> (60.9013, 26.555)
  arc A358 (62.9449, 27.9959) -> (62.9399, 27.9959) centre (62.9424, 27.9959) ccw
  arc A359 (62.7249, 27.5014) -> (62.7299, 27.5014) centre (62.7274, 27.5014) ccw
  arc A360 (61.9499, 26.7723) -> (61.9449, 26.7723) centre (61.9474, 26.7723) ccw
  arc A361 (62.9449, 27.9959) -> (62.9399, 27.9959) centre (62.9424, 27.9959) ccw
  line L103 (61.6994, 26.6647) -> (61.9474, 26.7723)
  arc A362 (60.9038, 26.555) -> (60.8988, 26.555) centre (60.9013, 26.555) ccw
  line L104 (61.1714, 26.555) -> (61.4394, 26.5918)
  arc A363 (62.1759, 26.9127) -> (62.1809, 26.9127) centre (62.1784, 26.9127) ccw
  line L105 (59.1302, 27.9959) -> (59.2207, 27.7413)
  arc A364 (59.0069, 36.7578) -> (59.0119, 36.7578) centre (59.0094, 36.7578) ccw
  arc A365 (59.1327, 27.9959) -> (59.1277, 27.9959) centre (59.1302, 27.9959) ccw
  arc A366 (59.2232, 27.7413) -> (59.2182, 27.7413) centre (59.2207, 27.7413) ccw
  line L106 (59.0482, 36.6468) -> (59.0614, 36.53)
  arc A367 (59.0507, 36.6468) -> (59.0457, 36.6468) centre (59.0482, 36.6468) ccw
  arc A368 (59.0639, 36.53) -> (59.0589, 36.53) centre (59.0614, 36.53) ccw
  arc A369 (59.2232, 27.7413) -> (59.2182, 27.7413) centre (59.2207, 27.7413) ccw
  arc A370 (59.0549, 28.5204) -> (59.0599, 28.5204) centre (59.0574, 28.5204) ccw
  line L107 (59.345, 27.5014) -> (59.5008, 27.2807)
  line L108 (59.0752, 28.2604) -> (59.1302, 27.9959)
  arc A371 (60.6361, 26.5918) -> (60.6311, 26.5918) centre (60.6336, 26.5918) ccw
  arc A372 (59.0599, 28.5204) -> (59.0549, 28.5204) centre (59.0574, 28.5204) ccw
  arc A373 (59.1327, 27.9959) -> (59.1277, 27.9959) centre (59.1302, 27.9959) ccw
  arc A374 (60.1231, 26.7723) -> (60.1281, 26.7723) centre (60.1256, 26.7723) ccw
  line L109 (60.1256, 26.7723) -> (60.3735, 26.6647)
  arc A375 (62.8549, 27.7413) -> (62.8499, 27.7413) centre (62.8524, 27.7413) ccw
  line L110 (59.6852, 27.0832) -> (59.8948, 26.9127)
  arc A376 (62.9399, 27.9959) -> (62.9449, 27.9959) centre (62.9424, 27.9959) ccw
  arc A377 (59.8923, 26.9127) -> (59.8973, 26.9127) centre (59.8948, 26.9127) ccw
  arc A378 (59.0549, 28.5204) -> (59.0599, 28.5204) centre (59.0574, 28.5204) ccw
  arc A379 (60.376, 26.6647) -> (60.371, 26.6647) centre (60.3735, 26.6647) ccw
  arc A380 (60.1281, 26.7723) -> (60.1231, 26.7723) centre (60.1256, 26.7723) ccw
  arc A381 (59.8973, 26.9127) -> (59.8923, 26.9127) centre (59.8948, 26.9127) ccw
  arc A382 (59.1277, 27.9959) -> (59.1327, 27.9959) centre (59.1302, 27.9959) ccw
  line L111 (59.0574, 28.5204) -> (59.0752, 28.2604)
  arc A383 (59.2182, 27.7413) -> (59.2232, 27.7413) centre (59.2207, 27.7413) ccw
  arc A384 (59.8923, 26.9127) -> (59.8973, 26.9127) centre (59.8948, 26.9127) ccw
  arc A385 (59.0589, 28.53) -> (59.0639, 28.53) centre (59.0614, 28.53) ccw
  arc A386 (59.0639, 28.53) -> (59.0589, 28.53) centre (59.0614, 28.53) ccw
  arc A387 (59.1277, 27.9959) -> (59.1327, 27.9959) centre (59.1302, 27.9959) ccw
  arc A388 (59.0589, 36.53) -> (59.0639, 36.53) centre (59.0614, 36.53) ccw
  line L112 (59.2207, 27.7413) -> (59.345, 27.5014)
  arc A389 (59.3475, 27.5014) -> (59.3425, 27.5014) centre (59.345, 27.5014) ccw
  line L113 (59.0094, 36.7578) -> (59.0482, 36.6468)
  arc A390 (59.0589, 28.53) -> (59.0639, 28.53) centre (59.0614, 28.53) ccw
  arc A391 (59.4983, 27.2807) -> (59.5033, 27.2807) centre (59.5008, 27.2807) ccw
  arc A392 (59.4983, 27.2807) -> (59.5033, 27.2807) centre (59.5008, 27.2807) ccw
  arc A393 (59.6827, 27.0832) -> (59.6877, 27.0832) centre (59.6852, 27.0832) ccw
  arc A394 (59.5033, 27.2807) -> (59.4983, 27.2807) centre (59.5008, 27.2807) ccw
  arc A395 (59.0639, 28.53) -> (59.0589, 28.53) centre (59.0614, 28.53) ccw
  line L114 (59.8948, 26.9127) -> (60.1256, 26.7723)
  arc A396 (59.0457, 36.6468) -> (59.0507, 36.6468) centre (59.0482, 36.6468) ccw
  arc A397 (59.0639, 36.53) -> (59.0589, 36.53) centre (59.0614, 36.53) ccw
  line L115 (59.0574, 28.5204) -> (59.0614, 28.53)
  arc A398 (59.0589, 36.53) -> (59.0639, 36.53) centre (59.0614, 36.53) ccw
  arc A399 (59.6877, 27.0832) -> (59.6827, 27.0832) centre (59.6852, 27.0832) ccw
  arc A400 (59.6827, 27.0832) -> (59.6877, 27.0832) centre (59.6852, 27.0832) ccw
  arc A401 (59.0777, 28.2604) -> (59.0727, 28.2604) centre (59.0752, 28.2604) ccw
  arc A402 (59.0599, 28.5204) -> (59.0549, 28.5204) centre (59.0574, 28.5204) ccw
  arc A403 (59.8973, 26.9127) -> (59.8923, 26.9127) centre (59.8948, 26.9127) ccw
  arc A404 (59.3425, 27.5014) -> (59.3475, 27.5014) centre (59.345, 27.5014) ccw
  arc A405 (60.1281, 26.7723) -> (60.1231, 26.7723) centre (60.1256, 26.7723) ccw
  arc A406 (59.5033, 27.2807) -> (59.4983, 27.2807) centre (59.5008, 27.2807) ccw
  line L116 (59.0614, 28.53) -> (59.0614, 36.53)
  arc A407 (59.0119, 36.7578) -> (59.0069, 36.7578) centre (59.0094, 36.7578) ccw
  arc A408 (59.3425, 27.5014) -> (59.3475, 27.5014) centre (59.345, 27.5014) ccw
  arc A409 (59.2182, 27.7413) -> (59.2232, 27.7413) centre (59.2207, 27.7413) ccw
  arc A410 (59.3475, 27.5014) -> (59.3425, 27.5014) centre (59.345, 27.5014) ccw
  line L117 (58.5364, 37.055) -> (58.6532, 37.0418)
  arc A411 (1.5098, 36.986) -> (1.5148, 36.986) centre (1.5123, 36.986) ccw
  arc A412 (58.6507, 37.0418) -> (58.6557, 37.0418) centre (58.6532, 37.0418) ccw
  arc A413 (59.0727, 28.2604) -> (59.0777, 28.2604) centre (59.0752, 28.2604) ccw
  arc A414 (0.4274, 36.2627) -> (0.4324, 36.2627) centre (0.4299, 36.2627) ccw
  line L118 (1.5123, 36.986) -> (1.7721, 37.0377)
  arc A415 (59.0507, 36.6468) -> (59.0457, 36.6468) centre (59.0482, 36.6468) ccw
  arc A416 (2.0339, 37.055) -> (2.0389, 37.055) centre (2.0364, 37.055) ccw
  arc A417 (58.9444, 36.8573) -> (58.9494, 36.8573) centre (58.9469, 36.8573) ccw
  arc A418 (0.8062, 36.6365) -> (0.8012, 36.6365) centre (0.8037, 36.6365) ccw
  arc A419 (58.8612, 36.9405) -> (58.8662, 36.9405) centre (58.8637, 36.9405) ccw
  arc A420 (58.6557, 37.0418) -> (58.6507, 37.0418) centre (58.6532, 37.0418) ccw
  arc A421 (1.0264, 36.7837) -> (1.0214, 36.7837) centre (1.0239, 36.7837) ccw
  arc A422 (58.7617, 37.003) -> (58.7667, 37.003) centre (58.7642, 37.003) ccw
  arc A423 (2.0339, 37.055) -> (2.0389, 37.055) centre (2.0364, 37.055) ccw
  line L119 (0.8037, 36.6365) -> (1.0239, 36.7837)
  arc A424 (1.0214, 36.7837) -> (1.0264, 36.7837) centre (1.0239, 36.7837) ccw
  line L120 (1.7721, 37.0377) -> (2.0364, 37.055)
  arc A425 (59.6877, 27.0832) -> (59.6827, 27.0832) centre (59.6852, 27.0832) ccw
  arc A426 (58.9494, 36.8573) -> (58.9444, 36.8573) centre (58.9469, 36.8573) ccw
  line L121 (58.9469, 36.8573) -> (59.0094, 36.7578)
  arc A427 (1.5098, 36.986) -> (1.5148, 36.986) centre (1.5123, 36.986) ccw
  arc A428 (59.0457, 36.6468) -> (59.0507, 36.6468) centre (59.0482, 36.6468) ccw
  line L122 (2.0364, 37.055) -> (58.5364, 37.055)
  arc A429 (58.9444, 36.8573) -> (58.9494, 36.8573) centre (58.9469, 36.8573) ccw
  line L123 (0.6045, 36.4619) -> (0.8037, 36.6365)
  arc A430 (1.7746, 37.0377) -> (1.7696, 37.0377) centre (1.7721, 37.0377) ccw
  line L124 (1.0239, 36.7837) -> (1.2615, 36.9009)
  arc A431 (58.5389, 37.055) -> (58.5339, 37.055) centre (58.5364, 37.055) ccw
  arc A432 (59.0119, 36.7578) -> (59.0069, 36.7578) centre (59.0094, 36.7578) ccw
  arc A433 (2.0389, 37.055) -> (2.0339, 37.055) centre (2.0364, 37.055) ccw
  arc A434 (59.0727, 28.2604) -> (59.0777, 28.2604) centre (59.0752, 28.2604) ccw
  arc A435 (58.5339, 37.055) -> (58.5389, 37.055) centre (58.5364, 37.055) ccw
  line L125 (0.4299, 36.2627) -> (0.6045, 36.4619)
  line L126 (58.6532, 37.0418) -> (58.7642, 37.003)
  arc A436 (60.1231, 26.7723) -> (60.1281, 26.7723) centre (60.1256, 26.7723) ccw
  arc A437 (59.0777, 28.2604) -> (59.0727, 28.2604) centre (59.0752, 28.2604) ccw
  arc A438 (58.6557, 37.0418) -> (58.6507, 37.0418) centre (58.6532, 37.0418) ccw
  arc A439 (59.0069, 36.7578) -> (59.0119, 36.7578) centre (59.0094, 36.7578) ccw
  arc A440 (60.371, 26.6647) -> (60.376, 26.6647) centre (60.3735, 26.6647) ccw
  arc A441 (0.602, 36.4619) -> (0.607, 36.4619) centre (0.6045, 36.4619) ccw
  arc A442 (58.6507, 37.0418) -> (58.6557, 37.0418) centre (58.6532, 37.0418) ccw
  arc A443 (0.8012, 36.6365) -> (0.8062, 36.6365) centre (0.8037, 36.6365) ccw
  arc A444 (58.9494, 36.8573) -> (58.9444, 36.8573) centre (58.9469, 36.8573) ccw
  arc A445 (1.0214, 36.7837) -> (1.0264, 36.7837) centre (1.0239, 36.7837) ccw
  arc A446 (58.7617, 37.003) -> (58.7667, 37.003) centre (58.7642, 37.003) ccw
  arc A447 (2.0389, 37.055) -> (2.0339, 37.055) centre (2.0364, 37.055) ccw
  line L127 (58.8637, 36.9405) -> (58.9469, 36.8573)
  arc A448 (58.8662, 36.9405) -> (58.8612, 36.9405) centre (58.8637, 36.9405) ccw
  arc A449 (1.5148, 36.986) -> (1.5098, 36.986) centre (1.5123, 36.986) ccw
  line L128 (1.2615, 36.9009) -> (1.5123, 36.986)
  arc A450 (1.259, 36.9009) -> (1.264, 36.9009) centre (1.2615, 36.9009) ccw
  arc A451 (0.8062, 36.6365) -> (0.8012, 36.6365) centre (0.8037, 36.6365) ccw
  line L129 (59.5008, 27.2807) -> (59.6852, 27.0832)
  arc A452 (0.8012, 36.6365) -> (0.8062, 36.6365) centre (0.8037, 36.6365) ccw
  arc A453 (58.5339, 37.055) -> (58.5389, 37.055) centre (58.5364, 37.055) ccw
  arc A454 (1.7746, 37.0377) -> (1.7696, 37.0377) centre (1.7721, 37.0377) ccw
  line L130 (58.7642, 37.003) -> (58.8637, 36.9405)
  arc A455 (58.7667, 37.003) -> (58.7617, 37.003) centre (58.7642, 37.003) ccw
  arc A456 (1.264, 36.9009) -> (1.259, 36.9009) centre (1.2615, 36.9009) ccw
  arc A457 (58.8612, 36.9405) -> (58.8662, 36.9405) centre (58.8637, 36.9405) ccw
  arc A458 (0.607, 36.4619) -> (0.602, 36.4619) centre (0.6045, 36.4619) ccw
  arc A459 (1.7696, 37.0377) -> (1.7746, 37.0377) centre (1.7721, 37.0377) ccw
  arc A460 (1.5148, 36.986) -> (1.5098, 36.986) centre (1.5123, 36.986) ccw
  line L131 (0.2827, 19.2675) -> (0.4299, 19.0473)
  line L132 (0.2827, 36.0425) -> (0.4299, 36.2627)
  arc A461 (0.607, 18.8481) -> (0.602, 18.8481) centre (0.6045, 18.8481) ccw
  arc A462 (1.0264, 36.7837) -> (1.0214, 36.7837) centre (1.0239, 36.7837) ccw
  arc A463 (0.168, 19.5051) -> (0.163, 19.5051) centre (0.1655, 19.5051) ccw
  arc A464 (0.0262, 35.2943) -> (0.0312, 35.2943) centre (0.0287, 35.2943) ccw
  arc A465 (0.0829, 19.7559) -> (0.0779, 19.7559) centre (0.0804, 19.7559) ccw
  arc A466 (0.0312, 35.2943) -> (0.0262, 35.2943) centre (0.0287, 35.2943) ccw
  line L133 (0.0804, 35.5541) -> (0.1655, 35.8049)
  arc A467 (0.168, 35.8049) -> (0.163, 35.8049) centre (0.1655, 35.8049) ccw
  line L134 (0.1655, 19.5051) -> (0.2827, 19.2675)
  line L135 (0.0287, 20.0157) -> (0.0804, 19.7559)
  line L136 (0.0804, 19.7559) -> (0.1655, 19.5051)
  arc A468 (0.2802, 19.2675) -> (0.2852, 19.2675) centre (0.2827, 19.2675) ccw
  arc A469 (0.0262, 20.0157) -> (0.0312, 20.0157) centre (0.0287, 20.0157) ccw
  arc A470 (0.4274, 19.0473) -> (0.4324, 19.0473) centre (0.4299, 19.0473) ccw
  line L137 (0.0114, 20.28) -> (0.0287, 20.0157)
  arc A471 (58.8662, 36.9405) -> (58.8612, 36.9405) centre (58.8637, 36.9405) ccw
  line L138 (0.4299, 19.0473) -> (0.6045, 18.8481)
  line L139 (0.6045, 18.8481) -> (0.8037, 18.6735)
  arc A472 (0.163, 19.5051) -> (0.168, 19.5051) centre (0.1655, 19.5051) ccw
  arc A473 (58.7667, 37.003) -> (58.7617, 37.003) centre (58.7642, 37.003) ccw
  arc A474 (0.0262, 20.0157) -> (0.0312, 20.0157) centre (0.0287, 20.0157) ccw
  line L140 (0.0287, 35.2943) -> (0.0804, 35.5541)
  arc A475 (0.2852, 19.2675) -> (0.2802, 19.2675) centre (0.2827, 19.2675) ccw
  line L141 (0.0114, 35.03) -> (0.0287, 35.2943)
  arc A476 (0.4324, 36.2627) -> (0.4274, 36.2627) centre (0.4299, 36.2627) ccw
  arc A477 (0.0139, 35.03) -> (0.0089, 35.03) centre (0.0114, 35.03) ccw
  arc A478 (0.0779, 19.7559) -> (0.0829, 19.7559) centre (0.0804, 19.7559) ccw
  arc A479 (0.0139, 20.28) -> (0.0089, 20.28) centre (0.0114, 20.28) ccw
  arc A480 (0.4324, 36.2627) -> (0.4274, 36.2627) centre (0.4299, 36.2627) ccw
  arc A481 (0.4274, 36.2627) -> (0.4324, 36.2627) centre (0.4299, 36.2627) ccw
  arc A482 (0.2802, 36.0425) -> (0.2852, 36.0425) centre (0.2827, 36.0425) ccw
  arc A483 (0.168, 19.5051) -> (0.163, 19.5051) centre (0.1655, 19.5051) ccw
  arc A484 (0.2852, 19.2675) -> (0.2802, 19.2675) centre (0.2827, 19.2675) ccw
  arc A485 (0.4324, 19.0473) -> (0.4274, 19.0473) centre (0.4299, 19.0473) ccw
  line L142 (0.0114, 20.28) -> (0.0114, 35.03)
  arc A486 (0.0139, 35.03) -> (0.0089, 35.03) centre (0.0114, 35.03) ccw
  arc A487 (0.2852, 36.0425) -> (0.2802, 36.0425) centre (0.2827, 36.0425) ccw
  arc A488 (0.602, 36.4619) -> (0.607, 36.4619) centre (0.6045, 36.4619) ccw
  arc A489 (0.0829, 35.5541) -> (0.0779, 35.5541) centre (0.0804, 35.5541) ccw
  arc A490 (0.0779, 35.5541) -> (0.0829, 35.5541) centre (0.0804, 35.5541) ccw
  arc A491 (0.0089, 35.03) -> (0.0139, 35.03) centre (0.0114, 35.03) ccw
  arc A492 (0.163, 19.5051) -> (0.168, 19.5051) centre (0.1655, 19.5051) ccw
  line L143 (0.1655, 35.8049) -> (0.2827, 36.0425)
  arc A493 (0.2802, 36.0425) -> (0.2852, 36.0425) centre (0.2827, 36.0425) ccw
  arc A494 (1.259, 36.9009) -> (1.264, 36.9009) centre (1.2615, 36.9009) ccw
  arc A495 (1.264, 36.9009) -> (1.259, 36.9009) centre (1.2615, 36.9009) ccw
  arc A496 (0.2802, 19.2675) -> (0.2852, 19.2675) centre (0.2827, 19.2675) ccw
  arc A497 (0.4324, 19.0473) -> (0.4274, 19.0473) centre (0.4299, 19.0473) ccw
  arc A498 (0.4274, 19.0473) -> (0.4324, 19.0473) centre (0.4299, 19.0473) ccw
  arc A499 (0.0089, 20.28) -> (0.0139, 20.28) centre (0.0114, 20.28) ccw
  arc A500 (0.0312, 20.0157) -> (0.0262, 20.0157) centre (0.0287, 20.0157) ccw
  arc A501 (0.0829, 35.5541) -> (0.0779, 35.5541) centre (0.0804, 35.5541) ccw
  arc A502 (0.602, 18.8481) -> (0.607, 18.8481) centre (0.6045, 18.8481) ccw
  arc A503 (0.0829, 19.7559) -> (0.0779, 19.7559) centre (0.0804, 19.7559) ccw
  arc A504 (1.7696, 37.0377) -> (1.7746, 37.0377) centre (1.7721, 37.0377) ccw
  arc A505 (0.0312, 20.0157) -> (0.0262, 20.0157) centre (0.0287, 20.0157) ccw
  arc A506 (0.0779, 19.7559) -> (0.0829, 19.7559) centre (0.0804, 19.7559) ccw
  arc A507 (0.0089, 20.28) -> (0.0139, 20.28) centre (0.0114, 20.28) ccw
  arc A508 (58.5389, 37.055) -> (58.5339, 37.055) centre (58.5364, 37.055) ccw
  arc A509 (0.0312, 35.2943) -> (0.0262, 35.2943) centre (0.0287, 35.2943) ccw
  arc A510 (1.5148, 18.324) -> (1.5098, 18.324) centre (1.5123, 18.324) ccw
  arc A511 (0.607, 18.8481) -> (0.602, 18.8481) centre (0.6045, 18.8481) ccw
  arc A512 (1.259, 18.409) -> (1.264, 18.409) centre (1.2615, 18.409) ccw
  arc A513 (0.0089, 35.03) -> (0.0139, 35.03) centre (0.0114, 35.03) ccw
  arc A514 (3.5211, 18.189) -> (3.5261, 18.189) centre (3.5236, 18.189) ccw
  arc A515 (0.8012, 18.6735) -> (0.8062, 18.6735) centre (0.8037, 18.6735) ccw
  arc A516 (1.0214, 18.526) -> (1.0264, 18.526) centre (1.0239, 18.526) ccw
  line L144 (3.0364, 18.255) -> (3.0455, 18.259)
  arc A517 (1.7746, 18.272) -> (1.7696, 18.272) centre (1.7721, 18.272) ccw
  arc A518 (1.7746, 18.272) -> (1.7696, 18.272) centre (1.7721, 18.272) ccw
  arc A519 (0.0262, 35.2943) -> (0.0312, 35.2943) centre (0.0287, 35.2943) ccw
  line L145 (2.0364, 18.255) -> (3.0364, 18.255)
  line L146 (1.0239, 18.526) -> (1.2615, 18.409)
  arc A520 (2.0339, 18.255) -> (2.0389, 18.255) centre (2.0364, 18.255) ccw
  arc A521 (3.7523, 18.103) -> (3.7573, 18.103) centre (3.7548, 18.103) ccw
  arc A522 (3.0339, 18.255) -> (3.0389, 18.255) centre (3.0364, 18.255) ccw
  line L147 (1.7721, 18.272) -> (2.0364, 18.255)
  arc A523 (0.607, 36.4619) -> (0.602, 36.4619) centre (0.6045, 36.4619) ccw
  arc A524 (1.264, 18.409) -> (1.259, 18.409) centre (1.2615, 18.409) ccw
  line L148 (3.5236, 18.189) -> (3.7548, 18.103)
  arc A525 (3.043, 18.259) -> (3.048, 18.259) centre (3.0455, 18.259) ccw
  arc A526 (3.9689, 17.985) -> (3.9739, 17.985) centre (3.9714, 17.985) ccw
  arc A527 (3.5211, 18.189) -> (3.5261, 18.189) centre (3.5236, 18.189) ccw
  arc A528 (0.8062, 18.6735) -> (0.8012, 18.6735) centre (0.8037, 18.6735) ccw
  arc A529 (3.0389, 18.255) -> (3.0339, 18.255) centre (3.0364, 18.255) ccw
  arc A530 (3.048, 18.259) -> (3.043, 18.259) centre (3.0455, 18.259) ccw
  line L149 (0.8037, 18.6735) -> (1.0239, 18.526)
  arc A531 (1.5098, 18.324) -> (1.5148, 18.324) centre (1.5123, 18.324) ccw
  arc A532 (0.168, 35.8049) -> (0.163, 35.8049) centre (0.1655, 35.8049) ccw
  arc A533 (0.163, 35.8049) -> (0.168, 35.8049) centre (0.1655, 35.8049) ccw
  arc A534 (3.7523, 18.103) -> (3.7573, 18.103) centre (3.7548, 18.103) ccw